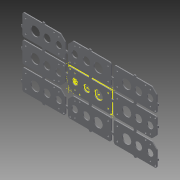
# Autodesk Inventor part: Granny Gearbox Input Plate Routing Template (9-up)
Saved by Autodesk Inventor 2015 (Build 190159000, 159)
## iProperties
Created: 2016-02-25
Part Number: Granny Gearbox Input Plate Routing Template (9-up)
Material: Generic
Document SubType Name: Modeling
Designer: sethbattis
Density: 1 g/cm^3
Appearance: Default
Author: sethbattis
Autodesk Inventor part; units mm, degrees
ref_plane "YZ Plane" through (0, 0, 0) normal (1, 0, 0) x (0, 1, 0)
ref_plane "XZ Plane" through (0, 0, 0) normal (0, 1, 0) x (-1, 0, 0)
ref_plane "XY Plane" through (0, 0, 0) normal (0, 0, 1) x (1, 0, 0)
derived "Granny Gearbox Input Plate.ipt"
feature "Solid1::Granny Gearbox Input Plate.ipt" [suppressed]
sketch "Shaft Alignment" plane through (0, 0, 0) normal (0, 0, 1) x (1, 0, 0)
  line L0 (-40.7035, -5.5985) -> (-0.0001, -11.1125) construction
  line L1 (-35.1409, -0.031) -> (-35.1353, -6.3528) construction
  line L2 (-11.1125, -0.0098) -> (-11.104, -9.6083) construction
  line L3 (0, 11.1125) -> (43.74, 13.9583) construction
  line L4 (-40.7035, -5.5985) -> (-46.2661, -5.5985) construction
  line L5 (-40.7035, -19.8733) -> (-46.2661, -19.8733) construction
  line L6 (-40.7035, 19.8015) -> (-46.2661, 19.8015) construction
  line L7 (-40.7035, 5.5267) -> (-46.2661, 5.5267) construction
  line L8 (-46.2661, 25.3641) -> (-46.2661, -25.4359) construction
  line L9 (-40.7035, 25.3641) -> (-40.7035, -25.4359) construction
  line L10 (-40.7035, -0.0359) -> (0, 0) construction
  line L11 (0, 0) -> (40.6908, 0) construction
  line L12 (11.1125, 0) -> (11.1125, 11.8355) construction
  line L13 (26.4033, 0) -> (26.4033, 12.8304) construction
  circle A0 centre (-40.7035, 25.3641) radius 5.5626
  circle A1 centre (-40.7035, -25.4359) radius 5.5626
  circle A2 centre (40.6908, 0) radius 14.2875
  circle A3 centre (0, 0) radius 11.1125
  circle A4 centre (-40.7035, -0.0359) radius 5.5626
  point P0 (-33.5787, -27.5177)
sketch "New Mounting Holes" plane through (0, 0, 0) normal (0, 0, 1) x (1, 0, 0)
  circle A0 centre (-40.7035, -0.0359) radius 31.75 construction
  circle A1 centre (40.6908, 0) radius 36.195 construction
  circle A2 centre (0, 0) radius 36.195 construction
  line L0 (-57.7242, 30.4609) -> (-55.8383, 30.4609) construction
  line L1 (-57.7242, 30.4609) -> (-57.7242, 28.575) construction
  circle A3 centre (-57.7242, 30.4609) radius 3.175
  circle A4 centre (-24.3812, -30.912) radius 3.175
  line L2 (-65.3633, -38.1) -> (-65.3633, 38.1) construction
  line L3 (87.0367, -38.1) -> (-65.3633, -38.1) construction
  line L4 (87.0367, 38.1) -> (87.0367, -38.1) construction
  line L5 (-65.3633, 38.1) -> (87.0367, 38.1) construction
  line L6 (-55.8383, 38.1) -> (-55.8383, -38.1) construction
  line L7 (-65.3633, 28.575) -> (87.0367, 28.575) construction
  line L8 (-65.3633, -28.575) -> (87.0367, -28.575) construction
  line L9 (77.5117, 38.1) -> (77.5117, -38.1) construction
  circle A5 centre (74.3367, 23.3553) radius 3.175
  circle A6 centre (74.3367, -23.3553) radius 3.175
sketch "Labels" plane through (0, 0, 0) normal (0, 0, 1) x (1, 0, 0)
  circle A0 centre (-40.7035, -0.0359) radius 5.5626
  circle A1 centre (-40.7035, 25.3641) radius 5.5626
  circle A2 centre (-40.7035, -25.4359) radius 5.5626
  circle A3 centre (0, 0) radius 11.1125
  circle A4 centre (40.6908, 0) radius 14.2875
  line L0 (-5.8677, 26.2224) -> (48.5566, 26.2224) construction
  line L1 (48.5566, 26.2224) -> (48.5566, 22.1963) construction
  line L2 (48.5566, 22.1963) -> (-5.8677, 22.1963) construction
  line L3 (-5.8677, 22.1963) -> (-5.8677, 26.2224) construction
sketch "Exterior" plane through (0, 0, 0) normal (0, 0, 1) x (1, 0, 0)
  line L0 (-65.3633, -17.4045) -> (-65.3633, 31.75)
  line L1 (-59.0133, 38.1) -> (80.6867, 38.1)
  line L2 (87.0367, 31.75) -> (87.0367, -31.75)
  line L3 (80.6867, -38.1) -> (-44.6678, -38.1)
  arc A0 (87.0367, 31.75) -> (80.6867, 38.1) centre (80.6867, 31.75) ccw
  arc A1 (80.6867, -38.1) -> (87.0367, -31.75) centre (80.6867, -31.75) ccw
  arc A2 (-59.0133, 38.1) -> (-65.3633, 31.75) centre (-59.0133, 31.75) ccw
  circle A3 centre (-40.7035, -0.0359) radius 31.75 construction
  line L4 (-63.5034, -21.8946) -> (-49.1579, -36.2401)
  line L5 (-65.3633, -38.1) -> (-65.3633, 38.1) construction
  line L6 (87.0367, -38.1) -> (-65.3633, -38.1) construction
  arc A4 (-49.1579, -36.2401) -> (-44.6678, -38.1) centre (-44.6678, -31.75) ccw
  arc A5 (-65.3633, -17.4045) -> (-63.5034, -21.8946) centre (-59.0133, -17.4045) ccw
  point P0 (87.0367, 38.1)
  point P1 (-65.3633, -20.0348)
  point P2 (-47.2981, -38.1)
sketch "Input Labels" plane through (0, 0, 0) normal (0, 0, 1) x (1, 0, 0)
  circle A0 centre (-40.7035, 25.3641) radius 2.667
  circle A1 centre (-40.7035, -0.0359) radius 9.525
  circle A2 centre (-40.7035, -25.4359) radius 2.667
  circle A3 centre (0, 0) radius 11.1125
  line L0 (-5.8677, 22.1963) -> (-5.8677, 26.2224) construction
  line L1 (-5.8677, 26.2224) -> (48.5566, 26.2224) construction
  line L2 (48.5566, 26.2224) -> (48.5566, 22.1963) construction
  line L3 (48.5566, 22.1963) -> (-5.8677, 22.1963) construction
  circle A4 centre (40.6908, 0) radius 14.2875
  line L4 (-5.8677, 26.2224) -> (45.7507, 26.2224) construction
  line L5 (45.7507, 26.2224) -> (45.7507, 22.1963) construction
  line L6 (45.7507, 22.1963) -> (-5.8677, 22.1963) construction
  line L7 (-5.8677, 22.1963) -> (-5.8677, 26.2224) construction
sketch "Sketch6" plane through (0, 0, 0) normal (0, 0, 1) x (1, 0, 0)
  line L0 (-63.5034, -21.8946) -> (-49.1579, -36.2401) projected
  line L1 (87.0367, -38.1) -> (-65.3633, -38.1) construction
  line L2 (87.0367, 38.1) -> (87.0367, -38.1) construction
  circle A0 centre (0, 0) radius 11.1125 projected
  circle A1 centre (40.6908, 0) radius 14.2875 projected
  circle A2 centre (-40.7035, 25.3641) radius 2.667 projected
  circle A3 centre (-40.7035, -0.0359) radius 9.525 projected
  circle A4 centre (-40.7035, -25.4359) radius 2.667 projected
  circle A5 centre (-24.3812, -30.912) radius 3.175 projected
  circle A6 centre (-57.7242, 30.4609) radius 3.175 projected
  circle A7 centre (74.3367, -23.3553) radius 3.175 projected
  line L3 (-57.4893, 36.576) -> (5.2204, 36.576)
  line L4 (85.5127, 30.226) -> (85.5127, 15.0813)
  line L5 (79.1627, -36.576) -> (19.5731, -36.576)
  line L6 (-65.3633, 38.1) -> (87.0367, 38.1) construction
  line L7 (-65.3633, -38.1) -> (-65.3633, 38.1) construction
  line L8 (-61.9794, -21.2634) -> (-48.5267, -34.7161)
  line L9 (-63.8393, -16.7732) -> (-63.8393, 0.7938)
  circle A8 centre (-40.7035, -0.0359) radius 11.049
  circle A9 centre (0, 0) radius 12.6365
  circle A10 centre (40.6908, 0) radius 15.8115
  circle A11 centre (0, 0) radius 36.195 construction
  arc A12 (85.5127, 30.226) -> (79.1627, 36.576) centre (79.1627, 30.226) ccw
  arc A13 (-57.4893, 36.576) -> (-63.8393, 30.226) centre (-57.4893, 30.226) ccw
  arc A14 (-63.8393, -16.7732) -> (-61.9794, -21.2634) centre (-57.4893, -16.7732) ccw
  arc A15 (-48.5267, -34.7161) -> (-44.0365, -36.576) centre (-44.0365, -30.226) ccw
  arc A16 (79.1627, -36.576) -> (85.5127, -30.226) centre (79.1627, -30.226) ccw
  circle A17 centre (74.3367, 23.3553) radius 3.175 projected
  line L10 (9.1861, 40.3897) -> (9.2217, 41.3004)
  line L11 (9.2217, 41.3004) -> (15.5717, 41.3004)
  line L12 (15.5717, 41.3004) -> (15.5483, 40.6998)
  line L13 (9.2452, -40.6998) -> (9.2217, -41.3004)
  line L14 (9.2217, -41.3004) -> (15.5717, -41.3004)
  line L15 (15.5717, -41.3004) -> (15.6074, -40.3897)
  line L16 (89.4815, 4.7625) -> (90.2371, 4.7625)
  line L17 (90.2371, 4.7625) -> (90.2371, 11.1125)
  line L18 (90.2371, 11.1125) -> (89.4815, 11.1125)
  line L19 (-67.808, 4.7625) -> (-68.5637, 4.7625)
  line L20 (-68.5637, 4.7625) -> (-68.5637, 11.1125)
  line L21 (-68.5637, 11.1125) -> (-67.808, 11.1125)
  line L22 (19.514, 36.576) -> (79.1627, 36.576)
  line L23 (-63.8393, 15.0813) -> (-63.8393, 30.226)
  line L24 (5.2795, -36.576) -> (-44.0365, -36.576)
  line L25 (85.5127, 0.7938) -> (85.5127, -30.226)
  arc A18 (5.2204, 36.576) -> (9.1861, 40.3897) centre (5.2204, 40.5448) ccw
  arc A19 (15.5483, 40.6998) -> (19.514, 36.576) centre (19.514, 40.5448) ccw
  arc A20 (9.2452, -40.6998) -> (5.2795, -36.576) centre (5.2795, -40.5447) ccw
  arc A21 (19.5731, -36.576) -> (15.6074, -40.3897) centre (19.5731, -40.5447) ccw
  arc A22 (89.4815, 4.7625) -> (85.5127, 0.7938) centre (89.4815, 0.7938) ccw
  arc A23 (85.5127, 15.0813) -> (89.4815, 11.1125) centre (89.4815, 15.0813) ccw
  arc A24 (-67.808, 11.1125) -> (-63.8393, 15.0813) centre (-67.808, 15.0813) ccw
  arc A25 (-63.8393, 0.7938) -> (-67.808, 4.7625) centre (-67.808, 0.7938) ccw
  line L26 (9.2217, 41.3004) -> (9.2217, -41.3004) construction
  line L27 (-68.5637, 11.1125) -> (90.2371, 11.1125) construction
  point P0 (15.387, 36.576)
  dimension "d20" = 1.524
  dimension "d23" = 1.524
  dimension "d24" = 1.524
  dimension "d25" = 19.05
  dimension "d26" = 22.098
  dimension "d27" = 22.225
  dimension "d28" = 25.273
  dimension "d29" = 28.575
  dimension "d30" = 31.623
  dimension "d31" = 6.35
  dimension "d34" = 4.7244
  dimension "d35" = 4.7244
  dimension "d36" = 4.7244
  dimension "d38" = 1.524
  dimension "d39" = 3.9688
  dimension "d40" = 6.35
  constraints: 46 end point, 34 tangent, 26 point on circle, 16 centre point, 13 parallel, 11 equal radius, 6 perpendicular, 5 horizontal, 3 coincident, 3 equal length, 3 point on line, 1 collinear, 1 vertical
  measures "d20" distance between parallel lines of L3 L6
  measures "d23" distance between parallel lines of L2 L4
  measures "d24" distance between parallel lines of L0 L8
  measures "d25" diameter of A3
  measures "d26" diameter of A8
  measures "d27" diameter of A0
  measures "d28" diameter of A9
  measures "d29" diameter of A1
  measures "d30" diameter of A10
  measures "d31" radius of A12
  measures "d34" distance between parallel lines of L3 L11
  measures "d35" distance between parallel lines of L5 L14
  measures "d36" distance between parallel lines of L4 L17
  measures "d38" distance between parallel lines of L24 L1
  measures "d39" radius of A18
  measures "d40" distance of L10.end L11.end
extrude "Extrusion2" add sketch "Sketch6" along normal blind 3.175 contours L3 A18 L10 L11 L12 A19 L22 A12 L4 A23 L18 L17 L16 A22 L25 A16 L5 A21 L15 L14 L13 A20 L24 A15 L8 A14 L9 A25 L19 L20 L21 A24 L23 A13
mirror "Mirror1" about plane through (90.2371, 4.7625, 0) normal (1, 0, 0) of "Extrusion2"
mirror "Mirror2" about plane through (-68.5637, 11.1125, 0) normal (-1, 0, 0) of "Extrusion2"
mirror "Mirror3" about plane through (15.5717, 41.3004, 0) normal (0, 1, 0) of "Extrusion2", "Mirror1", "Mirror2"
mirror "Mirror4" about plane through (-146.3491, -41.3004, 0) normal (0, -1, 0) of "Extrusion2", "Mirror2", "Mirror1"
equation "\"d23\" = d20"
equation "\"d24\" = d20"
equation "\"d26\" = d25 + 2 * d20"
equation "\"d28\" = d27 + 2 * d20"
equation "\"d30\" = d29 + 2 * d20"
equation "\"d35\" = d34"
equation "\"d36\" = d34"
equation "\"d38\" = d20"
body "Solid1"
